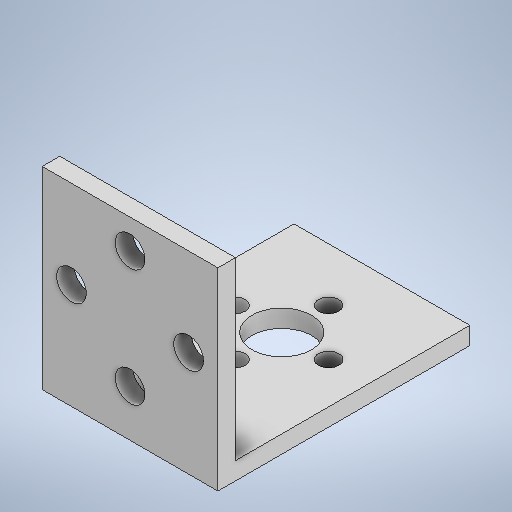
# Autodesk Inventor part: Leadnut Attachment
Saved by Autodesk Inventor 2025.2 (Build 292293000, 293)
## iProperties
Created: 2025-07-16
Part Number: Leadnut Attachment
Material: Generic
Document SubType Name: Modeling
Designer: Simon
Density: 1 g/cm^3
Appearance: Default
Author: Simon
Autodesk Inventor part; units mm, degrees
ref_plane "YZ Plane" through (0, 0, 0) normal (1, 0, 0) x (0, 1, 0)
ref_plane "XZ Plane" through (0, 0, 0) normal (0, 1, 0) x (-1, 0, 0)
ref_plane "XY Plane" through (0, 0, 0) normal (0, 0, 1) x (1, 0, 0)
sketch "Sketch1" plane through (0, 0, 0) normal (0, 0, 1) x (1, 0, 0)
  line L0 (-15, -15) -> (15, -15)
  line L1 (15, -15) -> (15, 15)
  line L2 (15, 15) -> (-15, 15)
  line L3 (-15, 15) -> (-15, -15)
  line L4 (-15, -15) -> (15, 15) construction
  line L5 (15, -15) -> (-15, 15) construction
  line L6 (0, -10) -> (0, 10)
  line L7 (-10, 0) -> (10, 0)
  circle A0 centre (-10, 0) radius 2.55
  circle A1 centre (0, 10) radius 2.55
  circle A2 centre (10, 0) radius 2.55
  circle A3 centre (0, -10) radius 2.55
  line L8 (-15, -15) -> (15, -15)
  line L9 (15, -15) -> (15, -18)
  line L10 (15, -18) -> (-15, -18)
  line L11 (-15, -18) -> (-15, -15)
  point P0 (0, 0)
  dimension "d0" = 30
  dimension "d1" = 30
  dimension "d2" = 20
  dimension "d3" = 20
  dimension "d4" = 5.1
  dimension "d5" = 5.1
  dimension "d6" = 5.1
  dimension "d7" = 5.1
  dimension "d8" = 3
  constraints: 24 end point, 4 centre point, 4 coincident, 4 midpoint, 4 parallel, 3 perpendicular, 2 horizontal, 1 vertical
  measures "d0" distance of L2.end L1.end
  measures "d1" distance of L1.end L0.end
  measures "d2" distance of L6.start L6.end
  measures "d3" distance of L7.start L7.end
  measures "d4" diameter of A0
  measures "d5" diameter of A1
  measures "d6" diameter of A2
  measures "d7" diameter of A3
  measures "d8" distance of L8.end L9.end
extrude "Extrusion1" add sketch "Sketch1" along normal blind 3
extrude "Extrusion2" add sketch "Sketch1" against normal blind 40 contours L0 L9 L10 L11
sketch "Sketch2" plane through (-15, -15, 0) normal (0, 1, 0) x (1, 0, 0)
  line L0 (0, 0) -> (0, -3) projected
  line L1 (30, 0) -> (30, 40) projected
  line L2 (0, 0) -> (30, 0)
  line L3 (30, 0) -> (15, 0)
  line L4 (15, 0) -> (15, 22.896)
  circle A0 centre (15, 22.896) radius 5.1
  circle A1 centre (15, 22.896) radius 8
  circle A2 centre (15, 14.896) radius 1.75
  circle A3 centre (23, 22.896) radius 1.75
  circle A4 centre (15, 30.896) radius 1.75
  circle A5 centre (7, 22.896) radius 1.75
  point P0 (13.2605, 30.7046)
  point P1 (16.7395, 30.7046)
  dimension "d15" = 16
  dimension "d13" = 22.896
  dimension "d14" = 10.2
  dimension "d16" = 3.5
  dimension "d19" = 360
  constraints: 6 end point, 5 centre point, 2 coincident, 2 perpendicular, 1 collinear, 1 point on line, 12 other
  measures "d13" distance of L3.end L4.end
  measures "d14" diameter of A0
  measures "d16" diameter of A2
extrude "Extrusion3" cut sketch "Sketch2" against normal blind 40 contours A2 A1 L4 | L4 A1 A2 | A1 A2 L4 | L4 A2 A1 | A0 | A5 A1 | A1 A5 | A3 A1 | A1 A3 | A4 A1 | A1 A4
body "Solid1"
